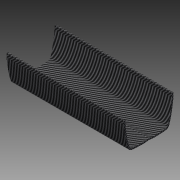
# Autodesk Inventor part: Cover
Saved by Autodesk Inventor 2016 (Build 200138000, 138)
## iProperties
Created: 2015-06-09
Part Number: Cover
Material: CFRP
Document SubType Name: Modeling
Designer: Yann
Density: 1.43 g/cm^3
Appearance: Carbon Fiber
Author: Yann
Autodesk Inventor part; units mm, degrees
ref_plane "YZ Plane" through (0, 0, 0) normal (1, 0, 0) x (0, 1, 0)
ref_plane "XZ Plane" through (0, 0, 0) normal (0, 1, 0) x (-1, 0, 0)
ref_plane "XY Plane" through (0, 0, 0) normal (0, 0, 1) x (1, 0, 0)
sketch "Sketch1" plane through (0, 0, 0) normal (1, 0, 0) x (0, 1, 0)
  line L0 (0, 47.2251) -> (0, -28.5505) construction
  line L1 (32.5, 31.4) -> (34.5, 31.4) construction
  line L2 (34.5, 31.4) -> (34.5, 38.4)
  line L3 (34.5, 38.4) -> (32.5, 38.4)
  line L4 (32.5, 38.4) -> (32.5, 31.4)
  line L5 (34.5, 31.4) -> (33.2277, 17.9619) construction
  line L6 (33.2277, 17.9619) -> (29.2964, 0.488) construction
  line L7 (29.2964, 0.488) -> (27.8164, -4.3687) construction
  line L8 (27.8164, -4.3687) -> (20.0769, -4.3147) construction
  line L9 (20.0769, -4.3147) -> (2.5994, -5.5867) construction
  line L10 (2.5994, -5.5867) -> (1.8458, -4.0773) construction
  line L11 (1.8458, -4.0773) -> (0, -4.0773) construction
  spline S0 degree 4 poles (34.5, 31.4) (33.2277, 17.9619) (29.2964, 0.488) (27.8164, -4.3687) (20.0769, -4.3147) (2.5994, -5.5867) (1.8458, -4.0773) (0, -4.0773) knots 1 1 1 1 1 2 3 4 5 5 5 5 5
  line L12 (-32.5, 31.4) -> (-34.5, 31.4) construction
  line L13 (-34.5, 31.4) -> (-34.5, 38.4)
  line L14 (-34.5, 38.4) -> (-32.5, 38.4)
  line L15 (-32.5, 38.4) -> (-32.5, 31.4)
  line L16 (-34.5, 31.4) -> (-33.2277, 17.9619) construction
  line L17 (-33.2277, 17.9619) -> (-29.2964, 0.488) construction
  line L18 (-29.2964, 0.488) -> (-27.8164, -4.3687) construction
  line L19 (-27.8164, -4.3687) -> (-20.0769, -4.3147) construction
  line L20 (-20.0769, -4.3147) -> (-2.5994, -5.5867) construction
  line L21 (-2.5994, -5.5867) -> (-1.8458, -4.0773) construction
  line L22 (-1.8458, -4.0773) -> (0, -4.0773) construction
  spline S1 degree 4 poles (-34.5, 31.4) (-33.2277, 17.9619) (-29.2964, 0.488) (-27.8164, -4.3687) (-20.0769, -4.3147) (-2.5994, -5.5867) (-1.8458, -4.0773) (0, -4.0773) knots 1 1 1 1 1 2 3 4 5 5 5 5 5
  line L23 (-68.4509, 0) -> (68.4509, 0) construction
  spline S2 degree 5 poles (32.5, 31.4) (32.2375, 28.6535) (31.9303, 25.9113) (31.5771, 23.1744) (30.8983, 18.5502) (30.0734, 13.9501) (29.7094, 12.0709) (29.0746, 9.0273) (28.3466, 6.0054) (28.0494, 4.8482) (27.567, 3.0826) (26.9827, 1.347) (26.7587, 0.7537) (26.4079, -0.0976) (25.9075, -0.8644) (25.7381, -1.088) (25.3152, -1.4884) (24.7848, -1.7262) (24.5048, -1.8201) (23.7056, -2.0391) (22.8858, -2.1654) (22.3578, -2.2339) (21.0572, -2.3734) (19.7529, -2.4715) (18.9793, -2.5236) (17.2634, -2.6292) (15.5464, -2.7187) (14.6037, -2.7647) (12.7167, -2.8495) (10.8289, -2.9149) (9.8843, -2.9413) (8.2275, -2.9722) (6.5705, -2.9486) (5.8589, -2.9244) (4.7209, -2.8563) (3.5923, -2.7012) (3.1709, -2.6288) (2.2932, -2.4224) (1.4198, -2.2016) (0.9496, -2.1199) (0.4744, -2.0868) (0, -2.0863) knots 0 0 0 0 0 0 0.232113 0.232113 0.232113 0.393137 0.393137 0.393137 0.493615 0.493615 0.493615 0.547091 0.547091 0.547091 0.570512 0.570512 0.570512 0.595337 0.595337 0.595337 0.640142 0.640142 0.640142 0.705366 0.705366 0.705366 0.784777 0.784777 0.784777 0.864274 0.864274 0.864274 0.924172 0.924172 0.924172 0.960078 0.960078 0.960078 1 1 1 1 1 1
  spline S3 degree 5 poles (0, -2.0863) (-0.4744, -2.0868) (-0.9496, -2.1199) (-1.4198, -2.2016) (-2.2932, -2.4224) (-3.1709, -2.6288) (-3.5923, -2.7012) (-4.7209, -2.8563) (-5.8589, -2.9244) (-6.5705, -2.9486) (-8.2275, -2.9722) (-9.8843, -2.9413) (-10.8289, -2.9149) (-12.7167, -2.8495) (-14.6037, -2.7647) (-15.5464, -2.7187) (-17.2634, -2.6292) (-18.9793, -2.5236) (-19.7529, -2.4715) (-21.0572, -2.3734) (-22.3578, -2.2339) (-22.8858, -2.1654) (-23.7056, -2.0391) (-24.5048, -1.8201) (-24.7848, -1.7262) (-25.3152, -1.4884) (-25.7381, -1.088) (-25.9075, -0.8644) (-26.4079, -0.0976) (-26.7587, 0.7537) (-26.9827, 1.347) (-27.567, 3.0826) (-28.0494, 4.8482) (-28.3466, 6.0054) (-29.0746, 9.0273) (-29.7094, 12.0709) (-30.0734, 13.9501) (-30.8983, 18.5502) (-31.5771, 23.1744) (-31.9303, 25.9113) (-32.2375, 28.6535) (-32.5, 31.4) knots 0 0 0 0 0 0 0.039922 0.039922 0.039922 0.075828 0.075828 0.075828 0.135726 0.135726 0.135726 0.215223 0.215223 0.215223 0.294634 0.294634 0.294634 0.359858 0.359858 0.359858 0.404663 0.404663 0.404663 0.429488 0.429488 0.429488 0.452909 0.452909 0.452909 0.506385 0.506385 0.506385 0.606863 0.606863 0.606863 0.767887 0.767887 0.767887 1 1 1 1 1 1
  point P0 (0, 0)
  point P1 (24, 0)
  point P2 (-24, 0)
  point P3 (5, 0.0487)
  dimension "d0" = 24
  dimension "d3" = 2
  dimension "d7" = 5
  dimension "d8" = 7
  constraints: 16 end point, 11 symmetric about line, 2 perpendicular, 2 point on line, 1 collinear, 1 horizontal, 1 vertical, 13 other
  measures "d0" distance from line of L0 point (24, 0)
  measures "d3" distance between parallel lines of L2 L4
  measures "d7" distance from line of L0 point (5, 0.049)
  measures "d8" distance of L3.end L1.start
ref_plane "Work Plane1" through (75, 32.5, 31.4) normal (-1, 0, 0) x (0, 0, 1)
ref_plane "Work Plane2" through (-75, 32.5, 31.4) normal (1, 0, 0) x (0, 1, 0)
ref_plane "Work Plane3" through (-82, -34.5, 31.4) normal (1, 0, 0) x (0, 1, 0)
ref_plane "Work Plane4" through (82, -34.5, 31.4) normal (-1, 0, 0) x (0, 0, 1)
extrude "Extrusion1" add sketch "Sketch1" along normal mid plane 144
equation "\"d3\" = Cover_Thickness"
equation "\"d8\" = Heatsink_Thickness"
equation "\"d4\" = PowerPCB_Length + 2 * Interface_Thickness"
equation "\"Heatsink_Thickness\" = 7"
equation "\"Cover_Thickness\" = 2"
equation "\"Heatsink_Width\" = 65"
equation "\"PowerPCB_Minus_Height\" = 1.2"
equation "\"Interface_Thickness\" = 7"
equation "\"PowerPCB_Thickness\" = 3"
equation "\"PowerPCB_Plus_Height\" = 8"
equation "\"LogicPCB_Width\" = 55"
equation "\"LogicPCB_Thickness\" = 2"
equation "\"LogicPCB_Plus_Height\" = 8"
equation "\"HostPCB_Thickness\" = 1.2"
equation "\"HostPCB_Plus_Height\" = 8"
equation "\"PowerPCB_Length\" = 130"
body "Solid1"
